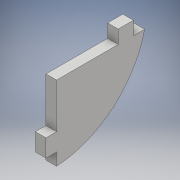
# Autodesk Inventor part: latéral
Saved by Autodesk Inventor 2017 (Build 210142000, 142)
## iProperties
Part Number: latéral
Material: Générique
Document SubType Name: Modeling
Designer: Thomas
Density: 1 g/cm^3
Appearance: Par défaut
Author: Thomas
Autodesk Inventor part; units mm, degrees
ref_plane "YZ Plane" through (0, 0, 0) normal (1, 0, 0) x (0, 1, 0)
ref_plane "XZ Plane" through (0, 0, 0) normal (0, 1, 0) x (-1, 0, 0)
ref_plane "XY Plane" through (0, 0, 0) normal (0, 0, 1) x (1, 0, 0)
sketch "Esquisse1" plane through (0, 0, 0) normal (1, 0, 0) x (0, 1, 0)
  line L0 (41, -0.4063) -> (49.6391, -0.4063)
  line L1 (0, -43.4063) -> (0, -33.4063)
  line L2 (49.6391, -0.4063) -> (41, -0.4063)
  line L3 (41, -0.4063) -> (41, -8.0057)
  line L4 (49.6391, -8.0057) -> (49.6391, -0.4063)
  line L5 (0, -33.4063) -> (6, -33.4063)
  line L6 (6, -33.4063) -> (6, -8.0057)
  line L7 (6, -43.4063) -> (6, -50.4063)
  line L8 (6, -43.4063) -> (0, -43.4063)
  line L9 (41, -8.0057) -> (6, -8.0057)
  line L10 (49.6391, -8.0057) -> (56, -8.0057)
  arc A0 (6, -50.4063) -> (56, -8.0057) centre (2.7397, 4.1194) ccw
  point P0 (0, 0)
  dimension "d2" = 35
  dimension "d3" = 33
  dimension "d4" = 6
  dimension "d5" = 6
  dimension "d6" = 10
  constraints: 22 end point, 3 perpendicular, 2 point on circle, 1 centre point, 1 horizontal, 1 parallel, 1 point on line
  measures "d2" distance between parallel lines of L6 L3
  measures "d3" distance between parallel lines of L5 L0
  measures "d4" distance between parallel lines of L1 L6
  measures "d5" distance between parallel lines of L1 L7
  measures "d6" distance between parallel lines of L8 L5
extrude "Extrusion1" add sketch "Esquisse1" along normal blind 6
